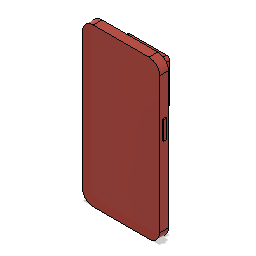
IPHONE_14P (Modeled) v9 (Autodesk Fusion 360 design; units mm, degrees)
Autodesk Fusion 360 part; units mm, degrees
sketch "Sketch1" plane through (0, 0, 0) normal (0, 0, 1) x (1, 0, 0)
  line L0 (36.05, 73.8) -> (-36.05, 73.8)
  line L1 (-36.05, 73.8) -> (-36.05, -73.8)
  line L2 (-36.05, -73.8) -> (36.05, -73.8)
  line L3 (36.05, -73.8) -> (36.05, 73.8)
  line L4 (36.05, 73.8) -> (-36.05, -73.8) construction
  line L5 (-36.05, 73.8) -> (36.05, -73.8) construction
  dimension "d1" = 72.1
  dimension "d2" = 147.6
  constraint horizontal L0
  constraint perpendicular L0 L1
  constraint parallel L0 L2
  constraint parallel L1 L3
  constraint coincident L4 origin
  constraint coincident L5 origin
  measures "d1" distance of L1.end L2.end
  measures "d2" distance of L0.end L1.end
extrude "Extrude1" add sketch "Sketch1" along normal blind 8 makes body 1
fillet "Fillet1" radius 10 4 edges at (-36.05, 73.8, 4) (36.05, 73.8, 4) (36.05, -73.8, 4) (-36.05, -73.8, 4) on bodies 1
sketch "Sketch2" plane through (0, 0, 0) normal (0, 0, -1) x (-1, 0, 0)
  arc A0 (26.05, -73.8) -> (36.05, -63.8) centre (26.05, -63.8) ccw
  line L0 (36.05, -63.8) -> (36.05, 63.8)
  arc A1 (36.05, 63.8) -> (26.05, 73.8) centre (26.05, 63.8) ccw
  line L1 (26.05, 73.8) -> (-26.05, 73.8)
  arc A2 (-26.05, 73.8) -> (-36.05, 63.8) centre (-26.05, 63.8) ccw
  line L2 (-36.05, 63.8) -> (-36.05, -63.8)
  arc A3 (-36.05, -63.8) -> (-26.05, -73.8) centre (-26.05, -63.8) ccw
  line L3 (-26.05, -73.8) -> (26.05, -73.8)
sketch "Sketch3" plane through (0, 0, 0) normal (0, 0, -1) x (1, 0, 0)
  line L0 (-7.95, -29.3) -> (32.55, -29.3)
  line L1 (32.55, -29.3) -> (32.55, -70.8)
  line L2 (32.55, -70.8) -> (-7.95, -70.8)
  line L3 (-7.95, -70.8) -> (-7.95, -29.3)
  line L4 (-7.95, -29.3) -> (32.55, -70.8) construction
  line L5 (32.55, -29.3) -> (-7.95, -70.8) construction
  line L6 (-26.05, -73.8) -> (26.05, -73.8)
  line L7 (36.05, -63.8) -> (36.05, 63.8)
  point P0 (12.3, -50.05)
  dimension "d9" = 40.5
  dimension "d10" = 41.5
  dimension "d18" = 3
  dimension "d19" = 3.5
  constraint horizontal L0
  constraint perpendicular L0 L1
  constraint parallel L0 L2
  constraint parallel L1 L3
  constraint coincident L4 P0
  constraint coincident L5 P0
  measures "d9" distance of L0.start L0.end
  measures "d10" distance of L0.start L2.end
  measures "d18" distance of L2 L6
  measures "d19" distance of L1 L7
extrude "Extrude2" add sketch "Sketch3" along normal blind 4.5 bodies 1
fillet "Fillet2" radius 3 4 edges at (32.55, 70.8, -2.25) (32.55, 29.3, -2.25) (-7.95, 70.8, -2.25) (-7.95, 29.3, -2.25) on bodies 1
sketch "Sketch4" plane through (36.05, 0, 0) normal (1, 0, 0) x (0, 0, -1)
  line L0 (-8, -63.8) -> (0, -63.8)
  line L1 (0, -63.8) -> (0, 63.8)
  line L2 (0, 63.8) -> (-8, 63.8)
  line L3 (-8, 63.8) -> (-8, -63.8)
  line L4 (4.5, 32.3) -> (4.5, 29.3)
  line L5 (4.5, 29.3) -> (0, 29.3)
  line L6 (4.5, 32.3) -> (4.5, 67.8)
  line L7 (4.5, 70.8) -> (4.5, 67.8)
  line L8 (0, 70.8) -> (4.5, 70.8)
  line L9 (-8, -73.8) -> (-8, -63.8)
  line L10 (0, -63.8) -> (0, -73.8)
  line L11 (0, -73.8) -> (-8, -73.8)
  line L12 (0, 29.3) -> (0, -63.8)
  line L13 (0, 73.8) -> (0, 70.8)
  line L14 (-8, 73.8) -> (0, 73.8)
  line L15 (-8, 63.8) -> (-8, 73.8)
  line L16 (-8, 63.8) -> (-8, -63.8)
  line L17 (-4, -63.8) -> (-4, 63.8) construction
  line L18 (-2.65, 9.6) -> (-5.35, 9.6)
  line L19 (-5.35, 9.6) -> (-5.35, 27.3)
  line L20 (-5.35, 27.3) -> (-2.65, 27.3)
  line L21 (-2.65, 27.3) -> (-2.65, 9.6)
  line L22 (-2.65, 9.6) -> (-5.35, 27.3) construction
  line L23 (-5.35, 9.6) -> (-2.65, 27.3) construction
  point P0 (-4, 18.45)
  dimension "d20" = 2.7
  dimension "d21" = 17.7
  dimension "d22" = 46.5
  constraint midpoint L0 L17.start
  constraint midpoint L2 L17.end
  constraint horizontal L18
  constraint perpendicular L18 L19
  constraint parallel L18 L20
  constraint parallel L19 L21
  constraint coincident L22 P0
  constraint coincident L23 P0
  constraint coincident L17 P0
  measures "d20" distance of L19.end L20.end
  measures "d21" distance of L18.end L19.end
  measures "d22" distance of L14 L20
extrude "Extrude3" add sketch "Sketch4" along normal blind 1 contours L18 L19 L20 L21 bodies 1
sketch "Sketch5" plane through (-36.05, 0, 0) normal (-1, 0, 0) x (0, 0, 1)
  line L0 (0, -63.8) -> (8, -63.8)
  line L1 (8, -63.8) -> (8, 63.8)
  line L2 (8, 63.8) -> (0, 63.8)
  line L3 (0, 63.8) -> (0, -63.8)
  line L4 (-4.5, 67.8) -> (-4.5, 70.8)
  line L5 (-4.5, 67.8) -> (-4.5, 32.3)
  line L6 (-4.5, 29.3) -> (-4.5, 32.3)
  line L7 (0, 29.3) -> (-4.5, 29.3)
  line L8 (-4.5, 70.8) -> (0, 70.8)
  line L9 (8, -73.8) -> (0, -73.8)
  line L10 (0, 70.8) -> (0, 73.8)
  line L11 (0, -63.8) -> (0, 29.3)
  line L12 (0, -73.8) -> (0, -63.8)
  line L13 (8, -63.8) -> (8, -73.8)
  line L14 (8, -63.8) -> (8, 63.8)
  line L15 (8, 73.8) -> (8, 63.8)
  line L16 (0, 73.8) -> (8, 73.8)
  line L17 (4, 63.8) -> (4, -63.8) construction
  line L18 (5.325, 35.05) -> (2.675, 35.05)
  line L19 (2.675, 35.05) -> (2.675, 23.85)
  line L20 (2.675, 23.85) -> (5.325, 23.85)
  line L21 (5.325, 23.85) -> (5.325, 35.05)
  line L22 (5.325, 35.05) -> (2.675, 23.85) construction
  line L23 (2.675, 35.05) -> (5.325, 23.85) construction
  line L24 (0, 22.35) -> (8, 22.35) construction
  line L25 (2.675, 9.65) -> (2.675, 20.85)
  line L26 (2.675, 20.85) -> (5.325, 20.85)
  line L27 (5.325, 9.65) -> (2.675, 9.65)
  line L28 (5.325, 20.85) -> (5.325, 9.65)
  point P0 (4, 29.45)
  dimension "d25" = 1.5
  dimension "d26" = 38.75
  dimension "d27" = 2.65
  dimension "d28" = 11.2
  constraint midpoint L2 L17.start
  constraint midpoint L0 L17.end
  constraint horizontal L18
  constraint perpendicular L18 L19
  constraint parallel L18 L20
  constraint parallel L19 L21
  constraint coincident L22 P0
  constraint coincident L23 P0
  constraint coincident L17 P0
  constraint coincident L11 L24.start
  constraint coincident L14 L24.end
  constraint perpendicular L14 L24
  constraint symmetric L18.start L24 L27.start
  constraint symmetric L18.end L24 L25.start
  constraint symmetric L19.end L24 L25.end
  constraint symmetric L20.end L24 L26.end
  measures "d25" distance of L20 L24
  measures "d26" distance of L16 L18
  measures "d27" distance of L19.end L20.end
  measures "d28" distance of L18.start L20.end
extrude "Extrude4" add sketch "Sketch5" along normal blind 1 contours L18 L19 L20 L21 | L25 L26 L27 L28 bodies 1
copy_body "CopyPasteBodies1" bodies 1 makes body 2
move_body "Move1" bodies 2 to x (1, 0, 0) y (0, 1, 0) z (0, 0, 1) at (0, 0, 0)
scale "Scale1" factors (1.006, 1.003, 1.04) about (-7.95, 32.3, 0) bodies 2
copy_body "CopyPasteBodies2" bodies 2 makes body 3
move_body "Move2" bodies 3 to x (-1, 0, 0) y (0, -1, 0) z (0, 0, 1) at (0.0744, -0.228, 0)
hidden bodies 1 3
named bodies: "IPHONE_14P", "IPHONE_14P_FIT", "IPHONE_14P_FIT REVERSED"
